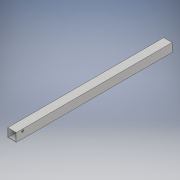
# Autodesk Inventor part: CLB_075_ScissorBase
Saved by Autodesk Inventor 2018.3 (Build 223284000, 284)
## iProperties
Created: 2020-02-18
Part Number: CLB_075_ScissorBase
Material: Generic
Document SubType Name: Modeling
Designer: 22perngrac
Density: 1 g/cm^3
Appearance: Default
Author: 22perngrac
Autodesk Inventor part; units mm, degrees
ref_plane "YZ Plane" through (0, 0, 0) normal (1, 0, 0) x (0, 1, 0)
ref_plane "XZ Plane" through (0, 0, 0) normal (0, 1, 0) x (-1, 0, 0)
ref_plane "XY Plane" through (0, 0, 0) normal (0, 0, 1) x (1, 0, 0)
sketch "Sketch1" plane through (0, 0, 0) normal (0, 0, 1) x (1, 0, 0)
  line L0 (0, 0) -> (25.4, 0)
  line L1 (25.4, 0) -> (25.4, 25.4)
  line L2 (25.4, 25.4) -> (0, 25.4)
  line L3 (0, 25.4) -> (0, 0)
  line L4 (1.5875, 23.8125) -> (23.8125, 23.8125)
  line L5 (23.8125, 23.8125) -> (23.8125, 1.5875)
  line L6 (23.8125, 1.5875) -> (1.5875, 1.5875)
  line L7 (1.5875, 1.5875) -> (1.5875, 23.8125)
  dimension "d0" = 25.4
  dimension "d1" = 1.5875
  constraints: 16 end point, 4 parallel, 3 perpendicular, 1 horizontal, 3 other
  measures "d0" distance of L1.end L2.end
  measures "d1" distance between parallel lines of L4 L2
extrude "Extrusion1" add sketch "Sketch1" along normal blind 463.55
sketch "Sketch2" plane through (25.4, 0, 0) normal (1, 0, 0) x (0, 0, -1)
  line L0 (0, 25.4) -> (-463.55, 25.4) projected
  line L1 (-463.55, 0) -> (-463.55, 25.4) projected
  line L2 (0, 0) -> (-463.55, 0) projected
  point P0 (-444.5, 19.304)
  dimension "d5" = 19.05
  dimension "d13" = 19.304
  measures "d5" distance from line of L1 point (-444.5, 19.304)
  measures "d13" distance from line of L2 point (-444.5, 19.304)
hole "Hole1" at (25.4, 19.304, 444.5) direction (-1, 0, 0) diameter 6.35 end through all
body "Solid1"
